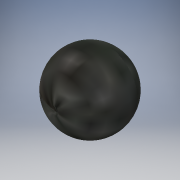
# Autodesk Inventor part: Parts_Ball_SBM-SUJ-6.5
Saved by Autodesk Inventor 2019.1 (Build 231200000, 200)
## iProperties
Created: 2018-08-21
Part Number: Parts_Ball_SBM-SUJ-6.5
Material: 鋼
Document SubType Name: Modeling
Designer: sktom
Density: 7.85 g/cm^3
Appearance: プレート
Author: sktom
Autodesk Inventor part; units mm, degrees
ref_plane "YZ Plane" through (0, 0, 0) normal (1, 0, 0) x (0, 1, 0)
ref_plane "XZ Plane" through (0, 0, 0) normal (0, 1, 0) x (-1, 0, 0)
ref_plane "XY Plane" through (0, 0, 0) normal (0, 0, 1) x (1, 0, 0)
sketch "スケッチ1" plane through (0, 0, 0) normal (0, 0, 1) x (1, 0, 0)
  circle A0 centre (0, 0) radius 2.25
  line L0 (-2.25, 0) -> (2.25, 0)
  dimension "d0" = 4.5
  constraints: 2 end point, 2 point on circle, 1 centre point, 1 coincident, 1 horizontal, 1 midpoint
  measures "d0" diameter of A0
revolve "回転1" add sketch "スケッチ1" angle 360 about axis through (-2.25, 0, 0) along (1, 0, 0) picked at (0.426, 0.6172) contours L0 A0
